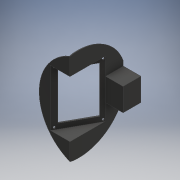
# Autodesk Inventor part: tapaVisor
Saved by Autodesk Inventor 2017 (Build 210142000, 142)
## iProperties
Part Number: tapaVisor
Material: Genérico
Document SubType Name: Modeling
Designer: Roberto
Density: 1 g/cm^3
Appearance: Valor por defecto
Author: Roberto
Autodesk Inventor part; units mm, degrees
ref_plane "YZ Plane" through (0, 0, 0) normal (1, 0, 0) x (0, 1, 0)
ref_plane "XZ Plane" through (0, 0, 0) normal (0, 1, 0) x (-1, 0, 0)
ref_plane "XY Plane" through (0, 0, 0) normal (0, 0, 1) x (1, 0, 0)
sketch "Boceto1" plane through (0, 0, 0) normal (0, 0, 1) x (1, 0, 0)
  line L0 (-5.810403, 0.016844) -> (-5.810403, 8.501968)
  line L1 (-9.300679, 8.404759) -> (-12.480588, 2.68706)
  line L2 (-19.216068, 2.88706) -> (-19.216068, 2.692644)
  line L3 (-9.475467, 8.501968) -> (-12.598208, 2.88706)
  line L4 (-12.480588, 2.68706) -> (-19.216068, 2.68706)
  line L5 (-12.598208, 2.88706) -> (-19.216068, 2.88706)
  line L6 (-12.137403, 2.892644) -> (-12.137403, 0.016844)
  line L7 (-12.137403, 0.016844) -> (-11.637403, 0.016844)
  line L8 (-11.637403, 0.016844) -> (-10.716403, 0.016844)
  line L9 (-10.716403, 0.016844) -> (-5.810403, 0.016844)
  line L10 (-9.475467, 8.501968) -> (-9.475467, 12.536799)
  line L11 (-9.300679, 8.404759) -> (-9.300679, 12.536799)
  line L12 (-9.475467, 12.536799) -> (-9.300679, 12.536799)
  line L13 (-9.300679, 12.536799) -> (-9.300679, 8.404759)
  line L14 (-9.300679, 8.404759) -> (-12.369358, 2.88706)
  line L15 (-12.480588, 2.68706) -> (-19.216068, 2.68706)
  line L16 (-19.216068, 2.68706) -> (-19.216068, 2.88706)
  line L17 (-19.216068, 2.88706) -> (-12.598208, 2.88706)
  line L18 (-12.486977, 3.08706) -> (-9.475467, 8.501968)
  line L19 (-9.475467, 8.501968) -> (-9.475467, 12.536799)
  line L20 (-9.475467, 12.536799) -> (-9.300679, 12.536799)
  line L21 (-9.300679, 12.536799) -> (-9.300679, 8.404759)
  line L22 (-9.300679, 8.404759) -> (-12.369358, 2.88706)
  line L23 (-12.480588, 2.68706) -> (-19.216068, 2.68706)
  line L24 (-19.216068, 2.68706) -> (-19.216068, 2.88706)
  line L25 (-19.216068, 2.88706) -> (-12.598208, 2.88706)
  line L26 (-12.486977, 3.08706) -> (-9.475467, 8.501968)
  line L27 (-9.475467, 8.501968) -> (-9.475467, 12.536799)
  line L28 (-9.475467, 12.536799) -> (-9.300679, 12.536799)
  line L29 (-9.475467, 8.501968) -> (-12.598208, 2.88706)
  line L30 (-12.598208, 2.88706) -> (-19.216068, 2.88706)
  line L31 (-19.216068, 2.88706) -> (-19.216068, 2.68706)
  line L32 (-19.216068, 2.68706) -> (-12.480588, 2.68706)
  line L33 (-12.480588, 2.68706) -> (-9.300679, 8.404759)
  constraints: 68 end point, 3 point on line, 2 perpendicular, 1 collinear, 1 horizontal, 1 vertical
extrude "Extrusión1" add sketch "Boceto1" along normal mid plane 15
sketch "Boceto4" plane through (0, 0, 0) normal (0, 0, 1) x (1, 0, 0)
  line L0 (-9.475467, 8.501968) -> (-12.486977, 3.08706)
  line L1 (-12.486977, 3.08706) -> (-9.475467, 8.501968)
  line L2 (-12.486977, 3.08706) -> (-9.475467, 8.501968)
  line L3 (-9.300679, 8.404759) -> (-12.369358, 2.88706)
  line L4 (-9.300679, 8.404759) -> (-12.369358, 2.88706)
  line L5 (-9.300679, 8.404759) -> (-12.369358, 2.88706)
  line L6 (-10.716403, 0.016844) -> (-5.810403, 0.016844)
  line L7 (-11.637403, 0.016844) -> (-10.716403, 0.016844)
  line L8 (-12.137403, 0.016844) -> (-11.637403, 0.016844)
  line L9 (-12.137403, 2.892644) -> (-12.137403, 0.016844)
  line L10 (-9.300679, 8.404759) -> (-9.300679, 12.536799)
  line L11 (-9.300679, 12.536799) -> (-9.300679, 8.404759)
  line L12 (-9.300679, 12.536799) -> (-9.300679, 8.404759)
  line L13 (-9.475467, 8.501968) -> (-9.475467, 12.536799)
  line L14 (-9.475467, 8.501968) -> (-9.475467, 12.536799)
  line L15 (-9.475467, 8.501968) -> (-9.475467, 12.536799)
  line L16 (-9.475467, 12.536799) -> (-9.300679, 12.536799)
  line L17 (-9.475467, 12.536799) -> (-9.300679, 12.536799)
  line L18 (-9.475467, 12.536799) -> (-9.300679, 12.536799)
  line L19 (-19.104838, 3.08706) -> (-19.104838, 2.892644)
  line L20 (-12.369358, 2.88706) -> (-19.104838, 2.88706)
  line L21 (-12.369358, 2.88706) -> (-19.104838, 2.88706)
  line L22 (-12.369358, 2.88706) -> (-19.104838, 2.88706)
  line L23 (-12.486977, 3.08706) -> (-19.104838, 3.08706)
  line L24 (-19.104838, 3.08706) -> (-12.486977, 3.08706)
  line L25 (-19.104838, 3.08706) -> (-12.486977, 3.08706)
  line L26 (-19.104838, 2.88706) -> (-19.104838, 3.08706)
  line L27 (-19.104838, 2.88706) -> (-19.104838, 3.08706)
  line L28 (-13.310403, 0.016844) -> (-13.004803, 0.016844)
  line L29 (-13.310403, 0.016844) -> (-13.004803, 0.016844)
  line L30 (-13.033659, 0.016844) -> (-13.310403, 0.016844)
  line L31 (-13.310403, 0.016844) -> (1.689597, 0.016844)
  line L32 (-13.033659, 0.016844) -> (-16.7627, 0.016844)
  line L33 (-16.7627, 21.947911) -> (-5.810403, 21.947911)
  line L34 (-16.7627, 21.947911) -> (-22.268428, 21.947911)
  line L35 (-22.268428, 21.947911) -> (-22.268428, 0.016844)
  line L36 (-22.268428, 0.016844) -> (-16.7627, 0.016844)
  line L37 (-12.137403, 0.016844) -> (-6.410403, 0.016844)
  line L38 (-6.410403, 0.016844) -> (-6.410403, -3.891215)
  arc A0 (-6.410403, 12.401858) -> (-10.015805, 11.328598) centre (-5.513991, 2.798096) ccw
  arc A1 (-9.948591, 11.363796) -> (-14.284428, 3.364792) centre (-6.224591, 4.170596) ccw
  line L39 (-13.633659, 0.016844) -> (-14.284428, 3.364792)
  line L40 (-14.284427, 3.364789) -> (-13.633659, 0.016844)
  line L41 (-6.410403, 12.644782) -> (-6.410403, 0.016844)
  line L42 (-6.410403, 21.947911) -> (-6.410403, 12.401858)
  line L43 (-6.410403, 12.401858) -> (-6.410403, 21.947911)
  line L44 (-6.410403, 21.947911) -> (-22.268428, 21.947911)
  line L45 (-22.268428, 21.947911) -> (-22.268428, 0.016844)
  line L46 (-22.268428, 0.016844) -> (-13.633659, 0.016844)
  line L47 (-13.633659, 0.016844) -> (-14.284427, 3.364789)
  point P0 (0, 0)
  point P1 (-13.310403, 0.016844)
  point P2 (-13.310403, 0.016844)
  point P3 (-13.310403, 0.016844)
  point P4 (-9.415805, 11.328598)
  dimension "d19" = 15
  dimension "d23" = 5.727
  constraints: 96 end point, 7 collinear, 5 horizontal, 5 point on circle, 4 perpendicular, 4 point on line, 2 centre point
  measures "d19" distance of L31.start L31.end
  measures "d23" distance of L9.end L37.end
revolve "Revolución2" cut sketch "Boceto4" angle 360 about axis through (-6.410403, 12.644782, 0) along (0, -1, 0) contours A0 A1 L39 L23 L19 L26 L20 L32 L36 L35 L34 L33 L42 L41 L10 L16 L13 | L13 L16 L10 A0 | L39 L20 L26 L19 L23
sketch "Boceto5" plane through (-9.475467, 8.501968, -5.55947) normal (-0.873936, 0.4860411, 0) x (0, 0, 1)
  line L0 (1.08947, -6.196) -> (10.02947, -6.196)
  line L1 (10.02947, 0) -> (1.08947, 0)
  line L2 (1.08947, 0) -> (10.02947, 0)
  line L3 (1.88947, -0.65) -> (9.22947, -0.65)
  line L4 (9.22947, -5.546) -> (1.88947, -5.546)
  arc A0 (1.43947, -6.096) -> (1.43947, -5.796) centre (1.43947, -5.946) ccw
  line L5 (1.43947, -6.096) -> (1.33947, -6.096)
  line L6 (1.33947, -5.796) -> (1.43947, -5.796)
  arc A1 (1.33947, -5.796) -> (1.33947, -6.096) centre (1.33947, -5.946) ccw
  line L7 (1.88947, -5.546) -> (1.88947, -0.65)
  line L8 (1.43947, -0.4) -> (1.33947, -0.4)
  line L9 (1.08947, 0) -> (1.08947, -6.196)
  arc A2 (1.43947, -0.4) -> (1.43947, -0.1) centre (1.43947, -0.25) ccw
  line L10 (1.33947, -0.1) -> (1.43947, -0.1)
  arc A3 (1.33947, -0.1) -> (1.33947, -0.4) centre (1.33947, -0.25) ccw
  arc A4 (9.67947, -5.796) -> (9.67947, -6.096) centre (9.67947, -5.946) ccw
  line L11 (9.77947, -6.096) -> (9.67947, -6.096)
  line L12 (9.67947, -5.796) -> (9.77947, -5.796)
  arc A5 (9.77947, -6.096) -> (9.77947, -5.796) centre (9.77947, -5.946) ccw
  line L13 (9.22947, -0.65) -> (9.22947, -5.546)
  line L14 (9.77947, -0.4) -> (9.67947, -0.4)
  arc A6 (9.67947, -0.1) -> (9.67947, -0.4) centre (9.67947, -0.25) ccw
  line L15 (10.02947, -6.196) -> (10.02947, 0)
  line L16 (10.02947, -6.196) -> (10.02947, 0)
  line L17 (9.67947, -0.1) -> (9.77947, -0.1)
  arc A7 (9.77947, -0.4) -> (9.77947, -0.1) centre (9.77947, -0.25) ccw
  point P0 (5.55947, -2.824709)
  point P1 (11.11894, 0)
  constraints: 36 end point, 16 point on circle, 8 centre point
extrude "Extrusión3" cut sketch "Boceto5" against normal blind 15 contours L3 L13 L4 L7 | L5 A1 L6 A0 | L8 A3 L10 A2 | L12 A5 L11 A4 | L14 A6 L17 A7
sketch "Boceto6" plane through (-9.475467, 8.501968, -5.911496) normal (-0.873936, 0.4860411, 0) x (0, 0, 1)
  line L0 (1.791496, -6.096) -> (1.691496, -6.096)
  line L1 (9.581496, -5.546) -> (2.241496, -5.546)
  line L2 (1.441496, -6.196) -> (10.381496, -6.196)
  line L3 (2.241496, -0.65) -> (9.581496, -0.65)
  line L4 (1.441496, 0) -> (10.381496, 0)
  line L5 (1.691496, -5.796) -> (1.791496, -5.796)
  arc A0 (1.691496, -5.796) -> (1.691496, -6.096) centre (1.691496, -5.946) ccw
  line L6 (2.241496, -5.546) -> (2.241496, -0.65)
  line L7 (1.791496, -0.4) -> (1.691496, -0.4)
  arc A1 (1.791496, -0.4) -> (1.791496, -0.1) centre (1.791496, -0.25) ccw
  line L8 (1.691496, -0.1) -> (1.791496, -0.1)
  line L9 (1.441496, 0) -> (1.441496, -6.196)
  arc A2 (1.791496, -6.096) -> (1.791496, -5.796) centre (1.791496, -5.946) ccw
  arc A3 (1.691496, -0.1) -> (1.691496, -0.4) centre (1.691496, -0.25) ccw
  line L10 (9.22947, -0.65) -> (9.22947, -5.546)
  arc A4 (10.031496, -0.1) -> (10.031496, -0.4) centre (10.031496, -0.25) ccw
  arc A5 (10.031496, -5.796) -> (10.031496, -6.096) centre (10.031496, -5.946) ccw
  line L11 (10.131496, -0.4) -> (10.031496, -0.4)
  line L12 (10.031496, -0.1) -> (10.131496, -0.1)
  line L13 (10.131496, -6.096) -> (10.031496, -6.096)
  line L14 (10.031496, -5.796) -> (10.131496, -5.796)
  arc A6 (10.131496, -0.4) -> (10.131496, -0.1) centre (10.131496, -0.25) ccw
  arc A7 (10.131496, -6.096) -> (10.131496, -5.796) centre (10.131496, -5.946) ccw
  line L15 (10.381496, -6.196) -> (10.381496, 0)
  line L16 (10.381496, -6.196) -> (10.381496, 0)
  line L17 (2.241496, -5.546) -> (2.241496, -0.65)
  line L18 (1.441496, 0) -> (-2.430485, 0)
  line L19 (-2.430485, 0) -> (-2.430485, -7.484569)
  line L20 (-2.430485, -7.484569) -> (1.441496, -7.484569)
  line L21 (1.441496, -7.484569) -> (1.441496, -6.196)
  line L22 (1.441496, 0) -> (1.441496, -7.484569)
  line L23 (10.381496, 0) -> (10.381496, -7.484569)
  line L24 (10.381496, 0) -> (13.44527, 0)
  line L25 (13.44527, 0) -> (13.44527, -7.484569)
  line L26 (13.44527, -7.484569) -> (10.381496, -7.484569)
  point P0 (5.911496, -2.824709)
  point P1 (5.55947, -2.824709)
  point P2 (11.470966, 0)
  constraints: 52 end point, 16 point on circle, 8 centre point, 5 perpendicular, 2 horizontal, 2 point on line, 1 collinear
extrude "Extrusión4" cut sketch "Boceto6" against normal blind 15 contours L21 L20 L19 L18 L9 | L15 L24 L25 L26 L23
sketch "Boceto8" plane through (-12.709438, 2.68706, 4.47) normal (0, -1, 0) x (1, 0, 0)
  line L0 (0.22885, 0) -> (0, 0)
  line L1 (0, 0) -> (0, 0.031688)
  arc A0 (0, 0.031688) -> (0, -8.971688) centre (6.299035, -4.47) ccw
  line L2 (0, -8.971688) -> (0, -8.94)
  line L3 (0, -8.94) -> (0.22885, -8.94)
  line L4 (0.22885, -8.94) -> (0.22885, 0)
  line L5 (-3.67192, 2.147568) -> (2.106513, 2.147568)
  line L6 (2.106513, 2.147568) -> (2.106513, -10.51185)
  line L7 (2.106513, -10.51185) -> (-3.67192, -10.51185)
  line L8 (-3.67192, -10.51185) -> (-3.67192, 2.147568)
  point P0 (12.709438, -4.47)
  constraints: 8 end point, 2 parallel, 1 horizontal, 1 perpendicular
extrude "Extrusión6" cut sketch "Boceto8" against normal blind 0.1 contours L4 L3 L2 A0 L1 L0 | L5 L6 L7 L8
sketch "Boceto9" plane through (-9.475467, 8.501968, -4.47) normal (-1, 0, 0) x (0, 0, 1)
  line L0 (0, 0) -> (0, -5.614907)
  line L1 (8.94, -5.614907) -> (8.94, 0)
  line L2 (0, 0) -> (0, 4.261177)
  line L3 (0, 4.261177) -> (-4.133561, 4.261177)
  line L4 (-4.133561, 4.261177) -> (-4.133561, -10.888559)
  line L5 (-4.133561, -10.888559) -> (0, -10.888559)
  line L6 (0, -10.888559) -> (0, 4.261177)
  line L7 (8.94, 0) -> (0, 0)
  line L8 (8.94, 0) -> (8.94, -10.888559)
  line L9 (8.94, -10.888559) -> (13.242794, -10.888559)
  line L10 (13.242794, -10.888559) -> (13.242794, 4.261177)
  line L11 (13.242794, 4.261177) -> (8.94, 4.261177)
  line L12 (8.94, 4.261177) -> (8.94, 0)
  point P0 (4.47, -8.501968)
  constraints: 20 end point, 6 perpendicular, 6 point on line, 1 collinear, 1 vertical
extrude "Extrusión7" cut sketch "Boceto9" along normal blind 10 and the other way blind 5
sketch "Boceto10" plane through (-12.779517, 2.88706, 4.47) normal (0, 0, 1) x (1, 0, 0)
  line L0 (0.023762, -0.1) -> (0.354544, -0.1)
  line L1 (3.478838, 5.517699) -> (0.354544, -0.1)
  line L2 (3.478838, 7.221802) -> (3.478838, 5.517699)
  spline S0 degree 6 poles (3.304051, 7.130422) (3.33296, 7.146097) (3.361959, 7.161594) (3.391048, 7.176914) (3.420225, 7.192056) (3.449489, 7.207019) (3.478838, 7.221802) knots 0 0 0 0 0 0 0 1 1 1 1 1 1 1
  line L3 (3.304051, 5.614907) -> (3.304051, 7.130422)
  line L4 (0.18131, 0) -> (3.304051, 5.614907)
  line L5 (0, 0) -> (0.18131, 0)
  line L6 (0.023762, -0.1) -> (0, 0)
  line L7 (3.478838, 5.517699) -> (0.354544, -0.1)
  line L8 (0.18131, 0) -> (3.304051, 5.614907)
  line L9 (3.304051, 5.614907) -> (0.18131, 0)
  line L10 (0.023762, -0.1) -> (0.354544, -0.1)
  line L11 (0.354544, -0.1) -> (0.125695, -0.1)
  line L12 (3.304051, 5.614907) -> (3.478838, 5.929187)
  line L13 (0.18131, 0) -> (0.125695, -0.1)
  line L14 (3.478838, -0.1) -> (3.478838, 5.929187)
  line L15 (0.125695, -0.1) -> (3.478838, -0.1)
  point P0 (12.779517, -2.88706)
  constraints: 12 end point, 2 collinear, 2 horizontal, 1 point on line, 1 other
extrude "Extrusión8" add sketch "Boceto10" along normal blind 0.2 contours L13 L4 L12 L2 L1 L0 | L1 L14 L15 | L3 S0 L2 L12
sketch "Boceto11" plane through (-12.598208, 2.88706, -4.47) normal (0, 0, -1) x (-1, 0, 0)
  line L0 (-3.297528, -0.1) -> (-3.297528, 7.221802)
  spline S0 degree 6 poles (-3.297528, 7.221802) (-3.268179, 7.207019) (-3.238915, 7.192056) (-3.209738, 7.176914) (-3.180649, 7.161594) (-3.15165, 7.146097) (-3.122741, 7.130422) knots 0 0 0 0 0 0 0 1 1 1 1 1 1 1
  line L1 (-3.122741, 7.130422) -> (-3.122741, 5.614907)
  line L2 (-3.122741, 5.614907) -> (0.055615, -0.1)
  line L3 (0.055615, -0.1) -> (-3.297528, -0.1)
  point P0 (-12.598208, -2.88706)
  constraints: 1 other
extrude "Extrusión9" add sketch "Boceto11" along normal blind 0.2
sketch "Boceto12" plane through (-12.779517, 2.88706, 4.67) normal (0, 0, 1) x (1, 0, 0)
  line L0 (3.478838, -0.1) -> (3.478838, 7.221802)
  line L1 (3.304051, 7.130422) -> (3.304051, 5.614907)
  line L2 (3.304051, 5.614907) -> (0.125695, -0.1)
  line L3 (0.125695, -0.1) -> (3.478838, -0.1)
  line L4 (0.125695, -0.1) -> (3.478838, -0.1)
  line L5 (3.478838, -0.1) -> (3.478838, 0)
  line L6 (3.478838, -0.1) -> (3.478838, 5.517699)
  line L7 (3.304051, 0) -> (0.18131, 0)
  line L8 (0.125695, -0.1) -> (0.18131, 0)
  line L9 (0.125695, -0.1) -> (0.18131, 0)
  line L10 (3.304051, 7.130422) -> (3.304051, 0)
  line L11 (3.478838, 0) -> (3.478838, 7.221802)
  line L12 (3.478838, 7.221802) -> (3.304051, 7.130422)
  point P0 (12.779517, -2.88706)
  constraints: 14 end point, 3 collinear, 2 perpendicular, 2 point on line, 1 other
extrude "Extrusión10" add sketch "Boceto12" along normal blind 4 contours L3 L2 L7 L10 L1 L12 L0
sketch "Boceto13" plane through (-12.779517, 2.88706, 4.47) normal (0, 0, 1) x (1, 0, 0)
  line L0 (0.125695, -0.1) -> (0.18131, 0)
  line L1 (0, 0) -> (0.18131, 0)
  line L2 (0.023762, -0.1) -> (0, 0)
  line L3 (0.023762, -0.1) -> (0.125695, -0.1)
  point P0 (12.779517, -2.88706)
extrude "Extrusión11" add sketch "Boceto13" along normal blind 4.2
sketch "Boceto14" plane through (-12.598208, 2.88706, -4.67) normal (0, 0, -1) x (-1, 0, 0)
  line L0 (-3.297528, -0.1) -> (-3.297528, 7.221802)
  line L1 (-3.297528, 7.221802) -> (-3.122741, 7.130422)
  line L2 (-3.122741, 7.130422) -> (-3.122741, 0)
  line L3 (-3.122741, 0) -> (0.18131, 0)
  line L4 (0.18131, 0) -> (0.157548, -0.1)
  line L5 (0.157548, -0.1) -> (-3.297528, -0.1)
  point P0 (-12.598208, -2.88706)
extrude "Extrusión12" add sketch "Boceto14" along normal blind 4
sketch "Boceto15" plane through (-12.598208, 2.88706, -4.47) normal (0, 0, -1) x (-1, 0, 0)
  line L0 (0, 0) -> (0.055615, -0.1)
  line L1 (0.157548, -0.1) -> (0.055615, -0.1)
  line L2 (0.18131, 0) -> (0.157548, -0.1)
  line L3 (0, 0) -> (0.18131, 0)
  point P0 (-12.598208, -2.88706)
extrude "Extrusión13" add sketch "Boceto15" along normal blind 4
sketch "Boceto16" plane through (0, 0, 0) normal (0, 0, 1) x (1, 0, 0)
  line L0 (-9.300679, 8.404759) -> (-9.300679, 12.536799)
  line L1 (-9.300679, 12.536799) -> (-9.300679, 8.404759)
  line L2 (-9.300679, 12.536799) -> (-9.300679, 8.404759)
  line L3 (-9.475467, 8.501968) -> (-9.475467, 12.536799)
  line L4 (-9.475467, 8.501968) -> (-9.475467, 12.536799)
  line L5 (-9.475467, 8.501968) -> (-9.475467, 12.536799)
  line L6 (-9.475467, 12.536799) -> (-9.300679, 12.536799)
  line L7 (-9.475467, 12.536799) -> (-9.300679, 12.536799)
  line L8 (-9.475467, 12.536799) -> (-9.300679, 12.536799)
  line L9 (-9.475467, 8.501968) -> (-12.486977, 3.08706)
  line L10 (-12.486977, 3.08706) -> (-9.475467, 8.501968)
  line L11 (-12.486977, 3.08706) -> (-9.475467, 8.501968)
  line L12 (-9.300679, 8.404759) -> (-12.369358, 2.88706)
  line L13 (-9.300679, 8.404759) -> (-12.369358, 2.88706)
  line L14 (-9.300679, 8.404759) -> (-12.369358, 2.88706)
  line L15 (-12.486977, 3.08706) -> (-19.104838, 3.08706)
  line L16 (-19.104838, 3.08706) -> (-12.486977, 3.08706)
  line L17 (-19.104838, 3.08706) -> (-12.486977, 3.08706)
  line L18 (-19.104838, 3.08706) -> (-19.104838, 2.892644)
  line L19 (-19.104838, 2.88706) -> (-19.104838, 3.08706)
  line L20 (-19.104838, 2.88706) -> (-19.104838, 3.08706)
  line L21 (-12.369358, 2.88706) -> (-19.104838, 2.88706)
  line L22 (-12.369358, 2.88706) -> (-19.104838, 2.88706)
  line L23 (-12.369358, 2.88706) -> (-19.104838, 2.88706)
  line L24 (-10.716403, 0.016844) -> (-5.810403, 0.016844)
  line L25 (-12.137403, 2.892644) -> (-12.137403, 0.016844)
  line L26 (-12.137403, 0.016844) -> (-11.637403, 0.016844)
  line L27 (-11.637403, 0.016844) -> (-10.716403, 0.016844)
  line L28 (-13.310403, 0.016844) -> (1.689597, 0.016844)
  line L29 (-13.310403, 0.016844) -> (-13.004803, 0.016844)
  line L30 (-13.310403, 0.016844) -> (-13.004803, 0.016844)
  line L31 (-13.033659, 0.016844) -> (-13.310403, 0.016844)
  line L32 (-13.033659, 0.016844) -> (-16.7627, 0.016844)
  line L33 (-16.7627, 21.947911) -> (-5.810403, 21.947911)
  line L34 (-16.7627, 21.947911) -> (-22.268428, 21.947911)
  line L35 (-22.268428, 21.947911) -> (-22.268428, 0.016844)
  line L36 (-22.268428, 0.016844) -> (-16.7627, 0.016844)
  line L37 (-12.137403, 0.016844) -> (-6.410403, 0.016844)
  line L38 (-6.410403, 0.016844) -> (-6.410403, -3.891215)
  arc A0 (-9.948591, 11.363796) -> (-14.284428, 3.364792) centre (-6.224591, 4.170596) ccw
  arc A1 (-6.410403, 12.401858) -> (-10.015805, 11.328598) centre (-5.513991, 2.798096) ccw
  line L39 (-6.410403, 12.644782) -> (-6.410403, 0.016844)
  line L40 (-13.633659, 0.016844) -> (-14.284428, 3.364792)
  line L41 (-14.284427, 3.364789) -> (-13.633659, 0.016844)
  line L42 (-6.410403, 21.947911) -> (-6.410403, 12.401858)
  line L43 (-6.410403, 12.401858) -> (-6.410403, 21.947911)
  line L44 (-6.410403, 21.947911) -> (-22.268428, 21.947911)
  line L45 (-22.268428, 21.947911) -> (-22.268428, 0.016844)
  line L46 (-22.268428, 0.016844) -> (-13.633659, 0.016844)
  line L47 (-13.633659, 0.016844) -> (-14.284427, 3.364789)
  point P0 (0, 0)
  point P1 (0, 0)
  point P2 (-9.415805, 11.328598)
  point P3 (-13.310403, 0.016844)
  point P4 (-13.310403, 0.016844)
  point P5 (-13.310403, 0.016844)
  dimension "d49" = 15
  dimension "d50" = 5.727
  constraints: 96 end point, 7 collinear, 5 horizontal, 5 point on circle, 4 perpendicular, 4 point on line, 2 centre point
  measures "d49" distance of L29.start L28.end
  measures "d50" distance of L25.end L37.end
revolve "Revolución3" cut sketch "Boceto16" angle 360 about axis through (-6.410403, 12.644782, 0) along (0, -1, 0) contours A1 L3 L6 L0 | L0 L6 L3 A1 A0 L40 L15 L18 L19 L21 L32 L36 L35 L34 L33 L42 L39 | L21 L19 L18 L15 L40
sketch "Boceto17" plane through (-9.475467, 2.88706, 4.67) normal (-1, 0, 0) x (0, 0, 1)
  line L0 (0, 5.614907) -> (-9.34, 5.614907)
  line L1 (-6.47, 5.614907) -> (-3.07, 5.614907)
  line L2 (-3.07, 8.850291) -> (-6.47, 8.850291)
  line L3 (-3.095, 8.850291) -> (-3.195, 8.850291)
  line L4 (-6.47, 5.614907) -> (-6.47, 8.850291)
  line L5 (-3.07, 5.614907) -> (-3.07, 8.850291)
  line L6 (-6.47, 5.614907) -> (-6.17, 5.614907)
  line L7 (-6.17, 5.614907) -> (-6.17, 6.214907)
  line L8 (-3.07, 5.614907) -> (-3.57, 5.614907)
  line L9 (-3.57, 5.614907) -> (-3.57, 6.214907)
  line L10 (-6.17, 6.214907) -> (-3.57, 6.214907)
  point P0 (-4.67, -2.88706)
  point P1 (-6.445, 5.614907)
  point P2 (-3.095, 5.614907)
  dimension "d57" = 0.3
  dimension "d59" = 0.5
  constraints: 20 end point, 6 point on line, 3 perpendicular, 2 vertical
  measures "d57" distance of L1.start L6.end
  measures "d59" distance of L1.end L8.end
extrude "Extrusión14" cut sketch "Boceto17" against normal blind 4
sketch "Boceto18" plane through (-9.300679, 2.78706, 4.47) normal (1, 0, 0) x (0, 0, -1)
  line L0 (2.87, 5.714907) -> (2.87, 8.694111)
  line L1 (6.27, 8.644347) -> (6.27, 5.714907)
  line L2 (6.27, 5.714907) -> (2.87, 5.714907)
  line L3 (8.94, 5.617699) -> (0, 5.617699)
  line L4 (2.87, 8.694111) -> (2.77, 8.694111)
  line L5 (2.77, 8.694111) -> (2.77, 5.617699)
  line L6 (6.37, 5.617699) -> (2.77, 5.617699)
  line L7 (6.37, 5.617699) -> (6.37, 8.644347)
  line L8 (6.27, 8.644347) -> (6.37, 8.644347)
  line L9 (6.27, 8.644347) -> (6.27, 5.714907)
  line L10 (6.27, 5.714907) -> (9.14, 5.714907)
  line L11 (6.27, 5.714907) -> (2.87, 5.714907)
  line L12 (2.87, 5.714907) -> (2.87, 8.694111)
  line L13 (2.87, 8.694111) -> (2.77, 8.694111)
  line L14 (2.77, 8.694111) -> (2.77, 5.617699)
  line L15 (2.77, 5.617699) -> (6.37, 5.617699)
  line L16 (6.37, 5.617699) -> (6.37, 8.644347)
  point P0 (4.47, -2.78706)
  dimension "d62" = 0.1
  constraints: 24 end point, 4 perpendicular, 3 collinear, 3 parallel, 2 point on line, 1 horizontal, 1 vertical
  measures "d62" distance of L0.end L4.end
extrude "Extrusión15" add sketch "Boceto18" along normal blind 2.8
sketch "Boceto19" plane through (-6.500679, 2.78706, 4.47) normal (1, 0, 0) x (0, 0, -1)
  line L0 (2.87, 8.694111) -> (2.77, 8.694111)
  line L1 (2.87, 8.694111) -> (2.87, 8.444111)
  line L2 (2.87, 8.617943) -> (2.87, 5.714907)
  line L3 (2.87, 8.444111) -> (1.830259, 8.444111)
  line L4 (1.830259, 8.444111) -> (1.830259, 9.344111)
  line L5 (1.830259, 9.344111) -> (8.03398, 9.344111)
  line L6 (8.03398, 9.344111) -> (8.03398, 8.444111)
  line L7 (8.03398, 8.444111) -> (2.87, 8.444111)
  point P0 (4.47, -2.78706)
  dimension "d66" = 0.25
  dimension "d67" = 0.9
  dimension "d68" = 0.9
  constraints: 12 end point, 3 perpendicular, 2 point on line, 1 collinear
  measures "d66" distance of L0.start L1.end
  measures "d67" distance of L3.end L4.end
  measures "d68" distance of L5.end L6.end
extrude "Extrusión16" cut sketch "Boceto19" against normal blind 4
sketch "Boceto20" plane through (-6.500679, 2.78706, 4.47) normal (1, 0, 0) x (0, 0, -1)
  line L0 (2.77, 8.444111) -> (2.77, 5.617699)
  line L1 (6.37, 5.617699) -> (6.37, 8.444111)
  line L2 (2.77, 5.617699) -> (6.37, 5.617699)
  line L3 (2.77, 5.617699) -> (2.77, 8.444111)
  line L4 (8.94, 5.617699) -> (6.37, 5.617699)
  line L5 (2.77, 8.444111) -> (6.37, 8.444111)
  line L6 (6.37, 8.444111) -> (6.37, 5.617699)
  line L7 (6.37, 5.617699) -> (2.77, 5.617699)
  line L8 (2.77, 5.617699) -> (2.77, 8.444111)
  point P0 (4.47, -2.78706)
  constraints: 8 end point, 2 parallel, 1 horizontal, 1 perpendicular
extrude "Extrusión17" add sketch "Boceto20" against normal blind 0.15
